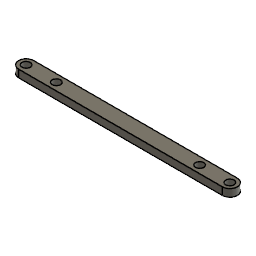
barra_soportes_giratorios (Autodesk Fusion 360 design; units mm, degrees)
part number: 2026-03-18-00-43-48-154
Autodesk Fusion 360 part; units mm, degrees
sketch "Boceto1" plane through (0, 0, 0) normal (0, 1, 0) x (1, 0, 0)
  line L0 (-67.4, -5) -> (67.4, -5)
  arc A0 (67.4, -5) -> (67.4, 5) centre (67.4, 0) ccw
  line L1 (67.4, 5) -> (-67.4, 5)
  arc A1 (-67.4, 5) -> (-67.4, -5) centre (-67.4, 0) ccw
  line L2 (-67.4, 0) -> (67.4, 0) construction
  circle A2 centre (-67.4, 0) radius 2.75
  circle A3 centre (67.4, 0) radius 2.75
  dimension "d1" = 10
  dimension "d2" = 134.8
  dimension "d3" = 5.5
  dimension "d4" = 5.5
  constraint tangent L0 A0
  constraint tangent A0 L1
  constraint parallel L0 L1
  constraint tangent L1 A1
  constraint tangent L0 A1
  constraint horizontal L2
  constraint midpoint L2 origin
  constraint concentric A1 A2
  constraint concentric A0 A3
  measures "d1" distance of L0 L1
  measures "d2" distance of A1.centre A0.centre
  measures "d3" diameter of A2
  measures "d4" diameter of A3
extrude "Extruir1" add sketch "Boceto1" along normal blind 5
sketch "Boceto2" plane through (0, 5, 0) normal (0, 1, 0) x (-1, 0, 0)
  circle A0 centre (-67.4, 0) radius 2.75
  circle A1 centre (67.4, 0) radius 2.75
  arc A2 (67.4, -5) -> (67.4, 5) centre (67.4, 0) ccw
  line L0 (67.4, 5) -> (-67.4, 5)
  arc A3 (-67.4, 5) -> (-67.4, -5) centre (-67.4, 0) ccw
  line L1 (-67.4, -5) -> (67.4, -5)
  circle A4 centre (47.4, 0) radius 2.75
  circle A5 centre (67.4, 0) radius 2.75
  line L2 (0, 0) -> (0, -16) construction
  circle A6 centre (-47.4, 0) radius 2.75
  dimension "d7" = 5.5
  dimension "d8" = 20
  constraint coincident L2.start origin
  constraint vertical L2
  constraint symmetric A4 L2 A6
  measures "d7" diameter of A4
  measures "d8" distance of A4.centre A1.centre
extrude "Extruir2" cut sketch "Boceto2" against normal blind 13 contours A4 | A6
